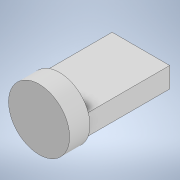
# Autodesk Inventor part: Bottom Pneumatics notch
Saved by Autodesk Inventor 2020 (Build 240168000, 168)
## iProperties
Created: 2021-01-30
Part Number: Bottom Pneumatics notch
Material: Generic
Document SubType Name: Modeling
Designer: magda
Density: 1 g/cm^3
Appearance: Default
Author: magda
Autodesk Inventor part; units mm, degrees
ref_plane "YZ Plane" through (0, 0, 0) normal (1, 0, 0) x (0, 1, 0)
ref_plane "XZ Plane" through (0, 0, 0) normal (0, 1, 0) x (-1, 0, 0)
ref_plane "XY Plane" through (0, 0, 0) normal (0, 0, 1) x (1, 0, 0)
sketch "Sketch1" plane through (0, 0, 0) normal (0, 0, 1) x (1, 0, 0)
  circle A0 centre (0, 0) radius 19.05
  dimension "d0" = 38.1
  constraints: 1 centre point, 1 coincident
  measures "d0" diameter of A0
extrude "Extrusion1" add sketch "Sketch1" along normal blind 12.7
sketch "Sketch2" plane through (0, 0, 0) normal (0, 0, -1) x (-1, 0, 0)
  circle A0 centre (0, 0) radius 19.05 projected
  line L0 (-17.9605, 6.35) -> (17.9605, 6.35)
  line L1 (17.9605, 6.35) -> (17.9605, -6.35)
  line L2 (17.9605, -6.35) -> (-17.9605, -6.35)
  line L3 (-17.9605, -6.35) -> (-17.9605, 6.35)
  dimension "d3" = 12.7
  dimension "d4" = 12.7
  constraints: 8 end point, 2 parallel, 2 point on circle, 1 horizontal, 1 perpendicular
  measures "d3" distance edge to line of A0 L0
  measures "d4" distance edge to line of A0 L2
extrude "Extrusion2" add sketch "Sketch2" along normal blind 50.8 contours L1 L2 L3 L0
body "Solid1"
